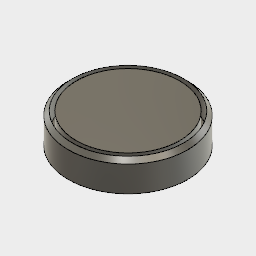
ANS0013_moving_top v1 (Autodesk Fusion 360 design; units mm, degrees)
Autodesk Fusion 360 part; units mm, degrees
sketch "Sketch1" plane through (0, 0, 0) normal (0, 1, 0) x (1, 0, 0)
  circle A0 centre (0, 0) radius 30
  dimension "d1" = 60
  measures "d1" diameter of A0
extrude "Extrude1" add sketch "Sketch1" along normal blind 15
sketch "Sketch2" plane through (0, 15, 0) normal (0, 1, 0) x (-1, 0, 0)
  circle A0 centre (0, 0) radius 30
  circle A1 centre (0, 0) radius 28
  circle A2 centre (0, 0) radius 26
  dimension "d4" = 56
  dimension "d5" = 52
  measures "d4" diameter of A1
  measures "d5" diameter of A2
extrude "Extrude2" cut sketch "Sketch2" against normal blind 10 contours A1
sketch "Sketch3" plane through (0, 0, 0) normal (0, -1, 0) x (1, 0, 0)
  circle A0 centre (0, 0) radius 30
  line L0 (0, 0) -> (5, 0)
  line L1 (0, 0) -> (-5, 0)
  circle A1 centre (0, 0) radius 30
  line L2 (0, 5) -> (-0.133, -10.9673)
  line L3 (5, 0) -> (5, 29.5804)
  line L4 (5, 0) -> (5, -29.5804)
  line L5 (-5, 0) -> (-5, 29.5804)
  line L6 (-5, 0) -> (-5, -29.5804)
  circle A2 centre (0, 0) radius 28
  dimension "d8" = 5
  dimension "d9" = 5
  dimension "d10" = 56
  constraint parallel L0 L1
  constraint coincident A1
  constraint perpendicular L0 L3
  constraint vertical L3
  constraint vertical L4
  constraint vertical L5
  constraint vertical L6
  measures "d10" diameter of A2
extrude "Extrude3" cut sketch "Sketch3" against normal blind 3 contours L0 L1 L3 L5 A2 | L0 L1 L4 L6 A2
sketch "Sketch4" plane through (0, 3, 0) normal (0, -1, 0) x (1, 0, 0)
  line L0 (5, -27.55) -> (5, 27.55)
  arc A0 (5, 27.55) -> (-5, 27.55) centre (0, 0) ccw
  line L1 (-5, 27.55) -> (-5, -27.55)
  arc A1 (-5, -27.55) -> (5, -27.55) centre (0, 0) ccw
  line L2 (5, 26) -> (-5, 26)
  line L3 (-5, 26) -> (-5, -26)
  line L4 (-5, -26) -> (5, -26)
  line L5 (5, -26) -> (5, 26)
  line L6 (5, 26) -> (-5, -26) construction
  line L7 (-5, 26) -> (5, -26) construction
  dimension "d13" = 52
  dimension "d14" = 10
  constraint perpendicular L2 L3
  constraint parallel L2 L4
  constraint parallel L3 L5
  constraint horizontal L2
  constraint coincident L6
  constraint coincident L7
extrude "Extrude4" cut sketch "Sketch4" against normal blind 8 contours L0 L1 L2 L3 L4 L5
chamfer "Chamfer1" distance 2 angle 45 1 edges at (-27.9698, 15, 10.8485)
